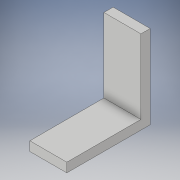
# Autodesk Inventor part: Bracket
Saved by Autodesk Inventor 2017 (Build 210142000, 142)
## iProperties
Created: 2019-03-26
Part Number: Bracket
Material: Generic
Document SubType Name: Modeling
Designer: mcgratta
Density: 1 g/cm^3
Appearance: Default
Author: mcgratta
Autodesk Inventor part; units mm, degrees
ref_plane "YZ Plane" through (0, 0, 0) normal (1, 0, 0) x (0, 1, 0)
ref_plane "XZ Plane" through (0, 0, 0) normal (0, 1, 0) x (-1, 0, 0)
ref_plane "XY Plane" through (0, 0, 0) normal (0, 0, 1) x (1, 0, 0)
sketch "Sketch1" plane through (0, 0, 0) normal (1, 0, 0) x (0, 1, 0)
  line L0 (0, 0) -> (28.575, 0)
  line L1 (28.575, 0) -> (28.575, 3.175)
  line L2 (28.575, 3.175) -> (3.175, 3.175)
  line L3 (3.175, 3.175) -> (3.175, 28.575)
  line L4 (3.175, 28.575) -> (0, 28.575)
  line L5 (0, 28.575) -> (0, 0)
  dimension "d0" = 25.4
  dimension "d1" = 28.575
  dimension "d2" = 3.175
  dimension "d3" = 25.4
  constraints: 12 end point, 5 perpendicular, 1 horizontal
  measures "d0" distance of L1.end L2.end
  measures "d1" distance of L0.start L0.end
  measures "d2" distance between parallel lines of L0 L2
  measures "d3" distance between parallel lines of L2 L4
extrude "Extrusion1" add sketch "Sketch1" along normal blind 12.7
body "Solid1"
